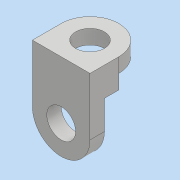
# Autodesk Inventor part: 8
Saved by Autodesk Inventor 2017 (Build 210142000, 142)
## iProperties
Part Number: 8
Material: 一般
Document SubType Name: Modeling
Designer: d8910
Density: 1 g/cm^3
Appearance: 預設
Author: d8910
Autodesk Inventor part; units mm, degrees
ref_plane "YZ Plane" through (0, 0, 0) normal (1, 0, 0) x (0, 1, 0)
ref_plane "XZ Plane" through (0, 0, 0) normal (0, 1, 0) x (-1, 0, 0)
ref_plane "XY Plane" through (0, 0, 0) normal (0, 0, 1) x (1, 0, 0)
sketch "草圖1" plane through (0, 0, 0) normal (0, 1, 0) x (-1, 0, 0)
  line L0 (10, 15) -> (-10, 15)
  line L1 (-10, 15) -> (-10, -5)
  line L2 (-10, -15) -> (10, -15) construction
  line L3 (10, -15) -> (10, -5) construction
  arc A0 (-10, -5) -> (10, -5) centre (0, -5) ccw
  line L4 (10, -5) -> (10, 15)
  line L5 (-10, -5) -> (-10, -15) construction
  circle A1 centre (0, -5) radius 5
  point P0 (0, 0)
  point P1 (10, 0)
  point P2 (0, 15)
  dimension "d0" = 30
  dimension "d1" = 20
  dimension "d2" = 5
  dimension "d3" = 10
  constraints: 12 end point, 5 parallel, 5 tangent, 2 centre point, 2 perpendicular, 2 point on circle, 1 coincident, 1 horizontal, 1 horizontal alignment, 1 midpoint, 1 vertical alignment
  measures "d0" distance of L2.end L0.start
  measures "d1" distance of L0.start L0.end
  measures "d2" distance of point (0, 0) A0.centre
  measures "d3" diameter of A1
extrude "擠出1" add sketch "草圖1" along normal blind 5
sketch "草圖2" plane through (-10, 0, 15) normal (0, 0, 1) x (1, 0, 0)
  line L0 (0, 0) -> (20, 0) construction
  line L1 (20, 0) -> (20, 5) construction
  line L2 (0, 5) -> (20, 5) construction
  line L3 (0, 0) -> (0, 5) construction
  line L4 (0, 5) -> (20, 5) projected
  line L5 (0, 5) -> (20, 5)
  line L6 (20, 5) -> (20, 10)
  line L7 (0, 10) -> (0, 5)
  arc A0 (20, 10) -> (0, 10) centre (10, 10) ccw
  circle A1 centre (10, 10) radius 5
  point P0 (10, 0)
  dimension "d6" = 5
  dimension "d7" = 10
  dimension "d8" = 10
  constraints: 6 end point, 2 centre point, 2 point on circle, 1 coincident, 1 horizontal, 1 parallel, 1 perpendicular, 1 tangent, 1 vertical alignment
  measures "d6" distance of L5.end L6.end
  measures "d7" radius of A0
  measures "d8" distance from line of L1 A0.centre
extrude "擠出2" add sketch "草圖2" against normal blind 5
sketch "草圖3" plane through (-10, 0, 10) normal (0, 0, -1) x (-1, 0, 0)
  line L0 (-10, 5) -> (-20, 5) projected
  circle A0 centre (-10, 10) radius 5 projected
  line L1 (0, 5) -> (-10, 5) projected
  line L2 (0, 5) -> (0, 10) projected
  arc A1 (0, 10) -> (-20, 10) centre (-10, 10) ccw projected
  line L3 (-20, 10) -> (-20, 5) projected
  line L4 (-20, 10) -> (-20, 5) projected
  line L5 (0, 5) -> (0, 10) projected
  line L6 (-20, 5) -> (0, 5)
  line L7 (0, 5) -> (0, 10)
  line L8 (0, 10) -> (-5, 10)
  line L9 (-20, 10) -> (-20, 5)
  line L10 (-15, 10) -> (-20, 10)
  line L11 (-5, 10) -> (-15, 10) construction
  point P0 (-10, 0)
  dimension "d11" = 5
  constraints: 12 end point, 4 parallel, 2 point on circle, 1 horizontal, 1 perpendicular, 1 point on line
  measures "d11" distance between parallel lines of L1 L8
extrude "擠出3" add sketch "草圖3" along normal blind 5 contours L0 L3 L10 A0 | A0 L8 L2 L1
